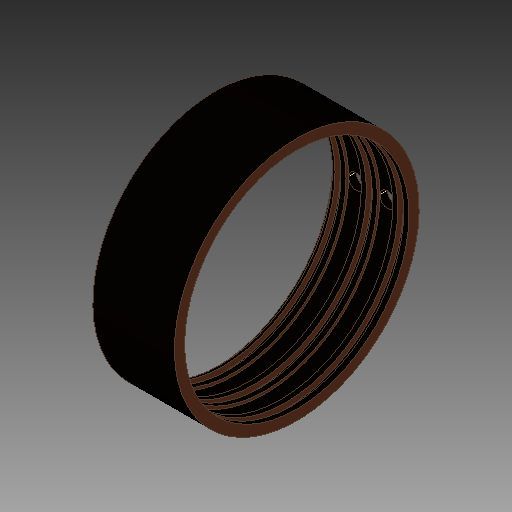
# Autodesk Inventor part: 1132_Outer RU Body_V1
Saved by Autodesk Inventor 2020 (Build 240168000, 168)
## iProperties
Created: 2017-08-07
Part Number: 1132_Outer RU Body_V1
Material: Bronze
Document SubType Name: Modeling
Designer: MPI
Density: 8.47 g/cm^3
Appearance: Bronze - Polished
Mass: 946.602 g
Surface Area: 650.63 cm^2
Volume: 111.759 cm^3
Author: MPI
Autodesk Inventor part; units mm, degrees
ref_plane "YZ Plane" through (0, 0, 0) normal (1, 0, 0) x (0, 1, 0)
ref_plane "XZ Plane" through (0, 0, 0) normal (0, 1, 0) x (-1, 0, 0)
ref_plane "XY Plane" through (0, 0, 0) normal (0, 0, 1) x (1, 0, 0)
sketch "Sketch1" plane through (0, 0, 0) normal (0, 0, 1) x (1, 0, 0)
  line L0 (14.8587, 0) -> (-14.8587, 0) construction
  line L1 (0, 69.8754) -> (46.0375, 69.8754) construction
  line L2 (6.8326, 71.4629) -> (16.3576, 71.4629) construction
  line L3 (16.3576, 71.4629) -> (16.3576, 68.2879) construction
  line L4 (16.3576, 68.2879) -> (6.8326, 68.2879) construction
  line L5 (6.8326, 68.2879) -> (6.8326, 71.4629) construction
  line L6 (6.8326, 71.4629) -> (16.3576, 68.2879) construction
  line L7 (16.3576, 71.4629) -> (6.8326, 68.2879) construction
  line L8 (0, 69.8754) -> (3.6576, 69.8754) construction
  line L9 (3.6576, 69.8754) -> (3.6576, 73.3298)
  line L10 (3.6576, 73.3298) -> (0, 73.3298)
  line L11 (0, 73.3298) -> (0, 69.8754)
  line L12 (11.5951, 69.8754) -> (11.5951, 71.4629) construction
  line L13 (0, 69.8754) -> (-1.5875, 69.8754)
  line L14 (-1.5875, 69.8754) -> (-1.5875, 73.0504)
  line L15 (-1.5875, 73.0504) -> (-4.7625, 73.0504)
  line L16 (-4.7625, 76.2) -> (46.0375, 76.2)
  line L17 (-4.7625, 73.0504) -> (-4.7625, 76.2)
  line L18 (19.5326, 69.8754) -> (19.5326, 73.3298)
  line L19 (19.5326, 73.3298) -> (23.1902, 73.3298)
  line L20 (23.1902, 73.3298) -> (23.1902, 69.8754)
  line L21 (21.3614, 69.8754) -> (21.3614, 73.3298) construction
  line L22 (35.8902, 71.4629) -> (26.3652, 71.4629) construction
  line L23 (26.3652, 71.4629) -> (26.3652, 68.2879) construction
  line L24 (26.3652, 68.2879) -> (35.8902, 68.2879) construction
  line L25 (35.8902, 68.2879) -> (35.8902, 71.4629) construction
  line L26 (35.8902, 71.4629) -> (26.3652, 68.2879) construction
  line L27 (26.3652, 71.4629) -> (35.8902, 68.2879) construction
  line L28 (42.7228, 69.8754) -> (39.0652, 69.8754) construction
  line L29 (39.0652, 69.8754) -> (39.0652, 73.3298)
  line L30 (39.0652, 73.3298) -> (42.7228, 73.3298)
  line L31 (42.7228, 73.3298) -> (42.7228, 69.8754)
  line L32 (31.1277, 69.8754) -> (31.1277, 71.4629) construction
  line L33 (46.0375, 69.8754) -> (46.0375, 76.2)
  line L34 (42.7228, 69.8754) -> (46.0375, 69.8754)
  line L35 (6.8326, 69.8754) -> (6.8326, 71.4629)
  line L36 (16.3576, 71.4629) -> (6.8326, 71.4629)
  line L37 (16.3576, 71.4629) -> (16.3576, 69.8754)
  line L38 (16.3576, 69.8754) -> (19.5326, 69.8754)
  line L39 (23.1902, 69.8754) -> (26.3652, 69.8754)
  line L40 (26.3652, 69.8754) -> (26.3652, 71.4629)
  line L41 (26.3652, 71.4629) -> (35.8902, 71.4629)
  line L42 (35.8902, 71.4629) -> (35.8902, 69.8754)
  line L43 (35.8902, 69.8754) -> (39.0652, 69.8754)
  line L44 (3.6576, 69.8754) -> (6.8326, 69.8754)
  point P0 (0, 0)
  point P1 (0, 0)
  dimension "d1" = 139.7508
  dimension "d3" = 3.6576
  dimension "d4" = 3.4544
  dimension "d5" = 3.175
  dimension "d6" = 1.5875
  dimension "d7" = 3.175
  dimension "d8" = 3.175
  dimension "d9" = 152.4
  dimension "d10" = 3.175
  dimension "d12" = 3.3147
  dimension "d13" = 1.5875
  dimension "d22" = 9.525
  dimension "d23" = 9.525
  dimension "d24" = 50.8
  dimension "d25" = 14.9098
  dimension "d27" = 19.6723
  dimension "d28" = 11.5951
  constraints: 90 end point, 14 symmetric about line, 11 midpoint, 7 perpendicular, 6 collinear, 5 horizontal, 3 point on line, 3 vertical, 2 parallel, 1 coincident, 1 vertical alignment
  measures "d1" diameter of L1 L0
  measures "d3" distance of L1.start L8.end
  measures "d4" distance of L8.end L9.end
  measures "d5" distance between parallel lines of L5 L9
  measures "d6" distance of L1.start L13.end
  measures "d7" distance of L13.end L14.end
  measures "d8" distance of L14.end L15.end
  measures "d9" diameter of L16 L0
  measures "d10" distance between parallel lines of L3 L18
  measures "d12" distance between parallel lines of L33 L31
  measures "d13" distance between parallel lines of L1 L2
  measures "d22" distance of L2.end L2.start
  measures "d23" distance of L25.end L23.start
  measures "d24" distance of L16.start L16.end
  measures "d25" distance from line of L33 L32.start
  measures "d27" distance between parallel lines of L33 L23
  measures "d28" distance between parallel lines of L35 L17
revolve "Revolution1" add sketch "Sketch1" angle 360 about axis through (14.8587, 0, 0) along (-1, 0, 0)
sketch "Sketch2" plane through (0, 0, 0) normal (0, 0, 1) x (1, 0, 0)
  line L0 (16.3576, -71.4629) -> (16.3576, 71.4629) projected
  line L1 (6.8326, -71.4629) -> (6.8326, 71.4629) projected
  line L2 (35.8902, -71.4629) -> (35.8902, 71.4629) projected
  line L3 (26.3652, -71.4629) -> (26.3652, 71.4629) projected
  line L4 (6.8326, 0) -> (35.8902, 0) construction
  line L5 (6.8326, 0) -> (16.3576, 0)
  line L6 (26.3652, 0) -> (35.8902, 0)
  point P0 (0, 0)
  point P1 (11.5951, 0)
  point P2 (31.1277, 0)
  constraints: 6 end point, 6 midpoint, 2 point on line, 1 collinear
hole "Hole1" at (11.5951, 0, 0) at (31.1277, 0, 0) direction (0, 0, -1) diameter 9.525 end through all
body "Solid1"
